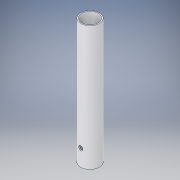
# Autodesk Inventor part: leg
Saved by Autodesk Inventor 2017 (Build 210142000, 142)
## iProperties
Created: 2016-09-16
Part Number: leg
Material: Generic
Document SubType Name: Modeling
Designer: Yeash
Density: 1 g/cm^3
Appearance: Default
Mass: 1634.46 g
Surface Area: 5201.25 cm^2
Volume: 1634.46 cm^3
Author: Yeash
Autodesk Inventor part; units mm, degrees
ref_plane "YZ Plane" through (0, 0, 0) normal (1, 0, 0) x (0, 1, 0)
ref_plane "XZ Plane" through (0, 0, 0) normal (0, 1, 0) x (-1, 0, 0)
sketch "Sketch1" plane through (0, 0, 0) normal (0, 1, 0) x (-1, 0, 0)
  circle A0 centre (0, 0) radius 57.15
  circle A1 centre (0, 0) radius 50.8
  dimension "d0" = 114.3
  dimension "d1" = 101.6
  constraints: 2 centre point, 2 coincident
  measures "d0" diameter of A0
  measures "d1" diameter of A1
extrude "Extrusion1" add sketch "Sketch1" along normal blind 762
ref_plane "Work Plane1" through (0, 0, 57.15) normal (0, 0, 1) x (1, 0, 0)
sketch "Sketch2" plane through (0, 0, 57.15) normal (0, 0, 1) x (1, 0, 0)
  line L0 (0, 0) -> (0, 101.6)
  circle A0 centre (0, 101.6) radius 12.7
  dimension "d4" = 101.6
  dimension "d5" = 25.4
  constraints: 2 end point, 1 centre point, 1 coincident, 1 vertical
  measures "d4" distance of L0.start L0.end
  measures "d5" diameter of A0
hole "Hole1" at (0, 101.6, 57.15) direction (0, 0, -1) diameter 25.4 end through all
body "Solid1"
